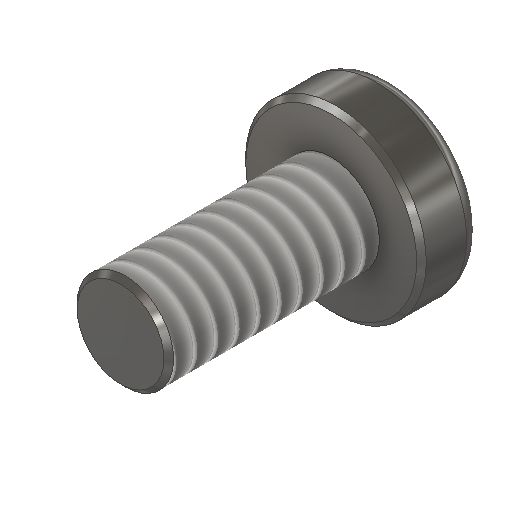
# Autodesk Inventor part: CNCT_STEEL_M1,6x3,5_Screw
Saved by Autodesk Inventor 2025 (Build 290162010, 162A)
## iProperties
Created: 2018-09-14
Part Number: CNCT_STEEL_M1,6x3,5_Screw
Material: Stainless Steel
Document SubType Name: Modeling
Designer: Andrzej
Density: 8 g/cm^3
Appearance: Steel - Polished
Mass: 0.0989484 g
Surface Area: 0.433607 cm^2
Volume: 0.0123685 cm^3
Author: Andrzej
Autodesk Inventor part; units mm, degrees
ref_plane "YZ Plane" through (0, 0, 0) normal (1, 0, 0) x (0, 1, 0)
ref_plane "XZ Plane" through (0, 0, 0) normal (0, 1, 0) x (-1, 0, 0)
ref_plane "XY Plane" through (0, 0, 0) normal (0, 0, 1) x (1, 0, 0)
sketch "Sketch1" plane through (0, 0, 0) normal (0, 0, 1) x (1, 0, 0)
  circle A0 centre (0, 0) radius 0.8
  circle A1 centre (0, 0) radius 1.5
  dimension "d0" = 1.6
  dimension "d1" = 3
  constraints: 2 centre point, 2 coincident
  measures "d0" diameter of A0
  measures "d1" diameter of A1
extrude "Extrusion1" add sketch "Sketch1" along normal blind 3.5 contours A0
extrude "Extrusion2" add sketch "Sketch1" against normal blind 1 contours A0 | A1
sketch "Sketch2" plane through (0, 0, -1) normal (0, 0, -1) x (-1, 0, 0)
  line L0 (-0.75, 0.433) -> (0, 0.866)
  line L1 (0, 0.866) -> (0.75, 0.433)
  line L2 (0.75, 0.433) -> (0.75, -0.433)
  line L3 (0.75, -0.433) -> (0, -0.866)
  line L4 (0, -0.866) -> (-0.75, -0.433)
  line L5 (-0.75, -0.433) -> (-0.75, 0.433)
  point P0 (0, 0)
  point P1 (0, 0)
  dimension "d6" = 1.5
  constraints: 12 end point, 1 coincident, 13 other
  measures "d6" distance between parallel lines of L2 L5
extrude "Extrusion3" cut sketch "Sketch2" against normal blind 0.8
fillet "Fillet1" radius 0.25 1 edges at (-1.5, 0, -1)
fillet "Fillet1" radius 0.1 6 edges at (0.375, 0.6495, -1) (0.75, 0, -1) (0.375, -0.6495, -1) (-0.375, -0.6495, -1) (-0.75, 0, -1) (-0.375, 0.6495, -1)
thread "Thread1" size "M1.6x0.35" class "6g" standard "ANSI Metric M Profile" full length
chamfer "Chamfer1" distance 0.08 angle 45 2 edges at (-0.8, 0, 3.5) (-1.5, 0, 0)
body "Solid1"
